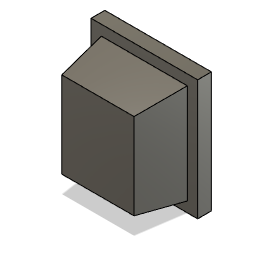
dictofun_button (Autodesk Fusion 360 design; units mm, degrees)
Autodesk Fusion 360 part; units mm, degrees
sketch "Sketch1" plane through (0, 0, 0) normal (0, 0, 1) x (1, 0, 0)
  line L0 (0, 0) -> (5, 0)
  line L1 (5, 0) -> (5, 5.8)
  line L2 (5, 5.8) -> (0, 5.8)
  line L3 (0, 5.8) -> (0, 0)
  dimension "d1" = 5
  dimension "d2" = 5.8
  constraint horizontal L0
  constraint vertical L1
  constraint horizontal L2
  constraint vertical L3
  constraint coincident L0.start L3.end
  measures "d1" distance of L0.start L0.end
  measures "d2" distance of L0.start L2.end
extrude "Extrude1" add sketch "Sketch1" along normal blind 3.5
sketch "Sketch2" plane through (0, 0, 0) normal (0, 0, -1) x (-1, 0, 0)
  line L0 (0, 0) -> (0, 5.8)
  line L1 (0, 5.8) -> (-5, 5.8)
  line L2 (-5, 5.8) -> (-5, 0)
  line L3 (-5, 0) -> (0, 0)
  line L4 (-4.4, 5.15) -> (-0.6, 5.15)
  line L5 (-0.6, 5.15) -> (-0.6, 0.65)
  line L6 (-0.6, 0.65) -> (-4.4, 0.65)
  line L7 (-4.4, 0.65) -> (-4.4, 5.15)
  dimension "d5" = 3.8
  dimension "d6" = 4.5
  dimension "d7" = 0.6
  dimension "d8" = 0.65
  constraint horizontal L4
  constraint vertical L5
  constraint horizontal L6
  constraint vertical L7
  measures "d5" distance of L4.start L4.end
  measures "d6" distance of L4.end L5.end
  measures "d7" distance of L2 L7
  measures "d8" distance of L1 L4
extrude "Extrude2" cut sketch "Sketch2" against normal blind 1.1 contours L4 L5 L6 L7
sketch "Sketch3" plane through (0, 0, 0) normal (0, 0, -1) x (-1, 0, 0)
  line L0 (-0.6, 5.15) -> (-0.6, 0.65)
  line L1 (-0.6, 0.65) -> (-4.4, 0.65)
  line L2 (-4.4, 0.65) -> (-4.4, 5.15)
  line L3 (-4.4, 5.15) -> (-0.6, 5.15)
  line L4 (0, 0) -> (0, 5.8)
  line L5 (0, 5.8) -> (-5, 5.8)
  line L6 (-5, 5.8) -> (-5, 0)
  line L7 (-5, 0) -> (0, 0)
  line L8 (-5.6, 6.4) -> (0.6, 6.4)
  line L9 (0.6, 6.4) -> (0.6, -0.6)
  line L10 (0.6, -0.6) -> (-5.6, -0.6)
  line L11 (-5.6, -0.6) -> (-5.6, 6.4)
  dimension "d11" = 0.6
  dimension "d12" = 0.6
  dimension "d13" = 0.6
  dimension "d14" = 0.6
  constraint horizontal L8
  constraint vertical L9
  constraint horizontal L10
  constraint vertical L11
  measures "d11" distance of L5 L8
  measures "d12" distance of L7 L10
  measures "d13" distance of L6 L11
  measures "d14" distance of L4 L9
extrude "Extrude3" add sketch "Sketch3" against normal blind 0.8 contours L8 L9 L10 L11
chamfer "Chamfer1" distance 0.4 distance2 2.7 4 edges at (5, 2.9, 3.5) (2.5, 5.8, 3.5) (0, 2.9, 3.5) (2.5, 0, 3.5) measured on face at (1.6667, 3.8667, 3.5) measured on face at (1.6667, 3.8667, 3.5) measured on face at (1.6667, 3.8667, 3.5) measured on face at (1.6667, 3.8667, 3.5)
